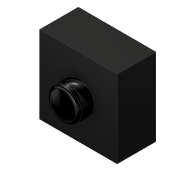
# Autodesk Inventor part: Power switch
Saved by Autodesk Inventor 2017 (Build 210142000, 142)
## iProperties
Created: 2016-08-05
Part Number: Power switch
Material: Generic
Document SubType Name: Modeling
Designer: ge937963
Density: 1 g/cm^3
Appearance: Default
Author: ge937963
Autodesk Inventor part; units mm, degrees
ref_plane "YZ Plane" through (0, 0, 0) normal (1, 0, 0) x (0, 1, 0)
ref_plane "XZ Plane" through (0, 0, 0) normal (0, 1, 0) x (-1, 0, 0)
ref_plane "XY Plane" through (0, 0, 0) normal (0, 0, 1) x (1, 0, 0)
sketch "Sketch1" plane through (0, 0, 0) normal (0, 0, 1) x (1, 0, 0)
  line L0 (0, 0) -> (13.0048, 0)
  line L1 (13.0048, 0) -> (13.0048, 13.0048)
  line L2 (13.0048, 13.0048) -> (0, 13.0048)
  line L3 (0, 13.0048) -> (0, 0)
  dimension "d0" = 13.0048
  dimension "d1" = 13.0048
  constraints: 8 end point, 2 parallel, 1 horizontal, 1 perpendicular
  measures "d0" distance of L2.end L0.start
  measures "d1" distance of L1.end L2.end
extrude "Extrusion1" add sketch "Sketch1" along normal blind 6.5
sketch "Sketch2" plane through (0, 0, 6.5) normal (0, 0, 1) x (1, 0, 0)
  circle A0 centre (6.5024, 6.5024) radius 2.65
  line L0 (13.0048, 0) -> (13.0048, 13.0048) projected
  line L1 (13.0048, 13.0048) -> (0, 13.0048) projected
  point P0 (0, 0)
  point P1 (13.0048, 6.5024)
  point P2 (6.5024, 13.0048)
  dimension "d4" = 5.3
  constraints: 2 midpoint, 1 centre point, 1 horizontal alignment, 1 vertical alignment
  measures "d4" diameter of A0
extrude "Extrusion2" add sketch "Sketch2" along normal blind 2.6
fillet "Fillet1" radius 0.508 1 edges at (3.8524, 6.5024, 9.1)
body "Solid1"
